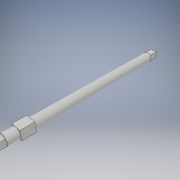
# Autodesk Inventor part: Arm Shaft
Saved by Autodesk Inventor 2017 (Build 210142000, 142)
## iProperties
Created: 2017-08-20
Part Number: Arm Shaft
Material: Generic
Document SubType Name: Modeling
Designer: Dale
Density: 1 g/cm^3
Appearance: Default
Author: Dale
## iProperties of the stored document Arm Shaft_3DPrint.ipt
Created: 2017-08-20
Part Number: Arm Shaft_3DPrint
Material: Generic
Document SubType Name: Modeling
Designer: Dale
Density: 1 g/cm^3
Appearance: Default
Author: Dale
Autodesk Inventor part; units mm, degrees
ref_plane "YZ Plane" through (0, 0, 0) normal (1, 0, 0) x (0, 1, 0)
ref_plane "XZ Plane" through (0, 0, 0) normal (0, 1, 0) x (-1, 0, 0)
ref_plane "XY Plane" through (0, 0, 0) normal (0, 0, 1) x (1, 0, 0)
sketch "Sketch1" plane through (0, 0, 0) normal (0, 0, 1) x (1, 0, 0)
  line L0 (-3.425, 3.425) -> (3.425, 3.425)
  line L1 (3.425, 3.425) -> (3.425, -3.425)
  line L2 (3.425, -3.425) -> (-3.425, -3.425)
  line L3 (-3.425, -3.425) -> (-3.425, 3.425)
  point P0 (0, 0)
  point P1 (0, 3.425)
  point P2 (3.425, 0)
  dimension "d0" = 6.85
  constraints: 8 end point, 2 midpoint, 2 parallel, 2 perpendicular, 1 horizontal, 1 horizontal alignment, 1 vertical alignment
  measures "d0" distance of L0.start L0.end
extrude "Left Lift Arm Drive" add sketch "Sketch1" along normal blind 11
sketch "Sketch2" plane through (0, 0, 0) normal (0, 0, -1) x (-1, 0, 0)
  circle A0 centre (0, 0) radius 4.8437
  point P0 (3.425, 3.425)
  dimension "d12" = 9.6874
  constraints: 1 coincident, 3 other
extrude "Left Lift Arm Support" add sketch "Sketch2" along normal blind 10
sketch "Sketch3" plane through (0, 0, -10) normal (0, 0, -1) x (-1, 0, 0)
  line L0 (-4.8437, 4.8437) -> (4.8437, 4.8437)
  line L1 (4.8437, 4.8437) -> (4.8437, -4.8437)
  line L2 (4.8437, -4.8437) -> (-4.8437, -4.8437)
  line L3 (-4.8437, -4.8437) -> (-4.8437, 4.8437)
  circle A0 centre (0, 0) radius 4.8437 projected
  point P0 (4.8437, 0)
  point P1 (0, 4.8437)
  dimension "d13" = 9.6874
  constraints: 8 end point, 2 midpoint, 2 parallel, 2 perpendicular, 2 vertical alignment, 1 horizontal, 1 horizontal alignment, 1 other
  measures "d13" distance of L0.start L0.end
extrude "Gear Drive" add sketch "Sketch3" along normal blind 12
sketch "Sketch4" plane through (0, 0, -22) normal (0, 0, -1) x (-1, 0, 0)
  circle A0 centre (0, 0) radius 4.8437
  line L0 (4.8437, 4.8437) -> (-4.8437, 4.8437) projected
  point P0 (0, 4.8437)
  constraints: 1 coincident, 1 midpoint, 1 vertical alignment, 2 other
extrude "Main Shaft" add sketch "Sketch4" along normal blind 138
sketch "Sketch5" plane through (0, 0, -160) normal (0, 0, -1) x (-1, 0, 0)
  line L0 (-3.425, 3.425) -> (3.425, 3.425)
  line L1 (3.425, 3.425) -> (3.425, -3.425)
  line L2 (3.425, -3.425) -> (-3.425, -3.425)
  line L3 (-3.425, -3.425) -> (-3.425, 3.425)
  circle A0 centre (0, 0) radius 4.8437 projected
  point P0 (3.425, 0)
  point P1 (0, 3.425)
  constraints: 8 end point, 2 midpoint, 2 parallel, 2 perpendicular, 1 horizontal, 1 horizontal alignment, 1 vertical alignment, 2 other
extrude "Right Lift Arm Drive" add sketch "Sketch5" along normal blind 11 contours L0 L1 L2 L3
sketch "Sketch6" plane through (0, 0, 11) normal (0, 0, 1) x (1, 0, 0)
  point P0 (0, 0)
  point P1 (0, 0)
  constraints: 1 coincident
hole "Left Cap Hole" at (0, 0, 11) direction (0, 0, -1) diameter 3 depth 8 tip angle 118 countersink diameter 4 countersink angle 90
sketch "Sketch7" plane through (0, 0, -171) normal (0, 0, -1) x (-1, 0, 0)
  circle A0 centre (0, 0) radius 1.5 projected
  constraints: 1 coincident
hole "Right Cap Hole" at (0, 0, -171) direction (0, 0, 1) diameter 3 depth 8 tip angle 118 countersink diameter 4 countersink angle 90
body "Solid1"
